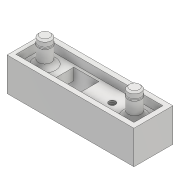
# Autodesk Inventor part: sipmHolder
Saved by Autodesk Inventor 2018 (Build 220112000, 112)
## iProperties
Created: 2017-05-10
Part Number: sipmHolder
Material: ABS Plastic
Document SubType Name: Modeling
Designer: sawaiz
Density: 1.06 g/cm^3
Appearance: Smooth - White
Author: sawaiz
Autodesk Inventor part; units mm, degrees
ref_plane "YZ Plane" through (0, 0, 0) normal (1, 0, 0) x (0, 1, 0)
sketch "Sketch1" plane through (0, 0, 0) normal (0, 0, 1) x (1, 0, 0)
  line L0 (-11.4, -3.5) -> (11.4, -3.5)
  line L1 (11.4, -3.5) -> (11.4, 3.5)
  line L2 (11.4, 3.5) -> (-11.4, 3.5)
  line L3 (-11.4, 3.5) -> (-11.4, -3.5)
  line L4 (-11.4, -3.5) -> (11.4, 3.5) construction
  line L5 (11.4, -3.5) -> (-11.4, 3.5) construction
  point P0 (0, 0)
  dimension "d0" = 22.8
  dimension "d1" = 7
  constraints: 12 end point, 2 midpoint, 2 parallel, 1 horizontal, 1 perpendicular
  measures "d0" distance of L2.end L1.end
  measures "d1" distance of L1.end L0.end
extrude "Extrusion1" add sketch "Sketch1" along normal mid plane 6
sketch "Sketch2" plane through (0, 0, 3) normal (0, 0, 1) x (1, 0, 0)
  line L0 (-5, 2.1) -> (-0.5, 2.1)
  line L1 (-0.5, 2.1) -> (-0.5, -2.1)
  line L2 (-0.5, -2.1) -> (-5, -2.1)
  line L3 (-5, -2.1) -> (-5, 2.1)
  line L4 (-5, 2.1) -> (-0.5, -2.1) construction
  line L5 (-0.5, 2.1) -> (-5, -2.1) construction
  line L6 (-11.4, 3.5) -> (-11.4, -3.5) projected
  line L7 (-2.75, 0) -> (-11.4, 0) construction
  point P0 (0, 0)
  dimension "d4" = 4.2
  dimension "d5" = 4.5
  dimension "d6" = 6.4
  constraints: 14 end point, 3 midpoint, 2 horizontal, 2 parallel, 1 perpendicular
  measures "d4" distance of L0.end L1.end
  measures "d5" distance of L0.start L0.end
  measures "d6" distance between parallel lines of L6 L3
extrude "Extrusion2" cut sketch "Sketch2" against normal through all
sketch "Sketch3" plane through (0, 0, 3) normal (0, 0, 1) x (1, 0, 0)
  line L0 (-5, -2.1) -> (-5, 2.1) projected
  line L1 (-5, 2.1) -> (-0.5, 2.1) projected
  line L2 (-0.5, 2.1) -> (-0.5, -2.1) projected
  line L3 (-0.5, -2.1) -> (-5, -2.1) projected
  line L4 (-11.4, -3.5) -> (11.4, -3.5) projected
  line L5 (11.4, -3.5) -> (11.4, 3.5) projected
  line L6 (11.4, 3.5) -> (-11.4, 3.5) projected
  line L7 (-11.4, 3.5) -> (-11.4, -3.5) projected
  line L8 (-10.7, -2.6) -> (10.5, -2.6)
  line L9 (10.5, -2.6) -> (10.5, 2.6)
  line L10 (10.5, 2.6) -> (-10.7, 2.6)
  line L11 (-10.7, 2.6) -> (-10.7, -2.6)
  line L12 (-10.7, -2.6) -> (10.5, 2.6) construction
  line L13 (10.5, -2.6) -> (-10.7, 2.6) construction
  dimension "d11" = 0.7
  dimension "d12" = 0.9
  dimension "d13" = 5.2
  dimension "d14" = 21.2
  constraints: 12 end point, 2 parallel, 1 horizontal, 1 perpendicular
  measures "d11" distance between parallel lines of L7 L11
  measures "d12" distance between parallel lines of L6 L10
  measures "d13" distance of L10.end L8.start
  measures "d14" distance of L9.end L10.end
extrude "Extrusion3" cut sketch "Sketch3" against normal blind 1.5 contours L11 L10 L9 L8
sketch "Sketch4" plane through (0, 0, -3) normal (0, 0, -1) x (-1, 0, 0)
  line L0 (-2.6, -2.1) -> (5, -2.1)
  line L1 (5, -2.1) -> (5, 2.1)
  line L2 (5, 2.1) -> (-2.6, 2.1)
  line L3 (-2.6, 2.1) -> (-2.6, -2.1)
  line L4 (-2.6, -2.1) -> (5, 2.1) construction
  line L5 (5, -2.1) -> (-2.6, 2.1) construction
  line L6 (5, 2.1) -> (5, -2.1) projected
  line L7 (5, -2.1) -> (0.5, -2.1) projected
  line L8 (0.5, -2.1) -> (0.5, 2.1) projected
  line L9 (0.5, 2.1) -> (5, 2.1) projected
  line L10 (-11.4, -3.5) -> (11.4, -3.5) projected
  line L11 (11.4, -3.5) -> (11.4, 3.5) projected
  line L12 (11.4, 3.5) -> (-11.4, 3.5) projected
  line L13 (-11.4, 3.5) -> (-11.4, -3.5) projected
  line L14 (0.5, 2.1) -> (5, 2.1) projected
  line L15 (5, -2.1) -> (0.5, -2.1) projected
  line L16 (5, 2.1) -> (5, -2.1) projected
  point P0 (0, 0)
  point P1 (1.2, 0)
  dimension "d17" = 14
  constraints: 12 end point, 3 collinear, 2 midpoint, 2 parallel, 1 horizontal, 1 perpendicular
  measures "d17" distance between parallel lines of L11 L3
extrude "Extrusion4" cut sketch "Sketch4" against normal blind 2.9 contours L3 L2 L8 L0 | L8 L2 L1 L0
sketch "Sketch5" plane through (0, 0, -3) normal (0, 0, -1) x (-1, 0, 0)
  line L0 (6.4, -2.1) -> (-6.5, -2.1)
  line L1 (-6.5, -2.1) -> (-6.5, 2.1)
  line L2 (-6.5, 2.1) -> (6.4, 2.1)
  line L3 (6.4, 2.1) -> (6.4, -2.1)
  line L4 (6.4, -2.1) -> (-6.5, 2.1) construction
  line L5 (-6.5, -2.1) -> (6.4, 2.1) construction
  line L6 (-2.6, 2.1) -> (5, 2.1) projected
  line L7 (5, -2.1) -> (-2.6, -2.1) projected
  line L8 (11.4, -3.5) -> (11.4, 3.5) projected
  point P0 (0, 0)
  point P1 (-0.05, 0)
  dimension "d20" = 12.9
  dimension "d21" = 5
  constraints: 12 end point, 2 collinear, 2 midpoint, 2 parallel, 1 horizontal, 1 perpendicular
  measures "d20" distance of L1.end L2.end
  measures "d21" distance between parallel lines of L8 L3
extrude "Extrusion5" cut sketch "Sketch5" against normal blind 2.4
sketch "Sketch6" plane through (0, 0, -3) normal (0, 0, -1) x (-1, 0, 0)
  line L0 (-6.5, 2.1) -> (6.4, 2.1) projected
  line L1 (6.4, 2.1) -> (6.4, -2.1) projected
  line L2 (6.4, -2.1) -> (-6.5, -2.1) projected
  line L3 (-6.5, -2.1) -> (-6.5, 2.1) projected
  line L4 (-11.4, -3.5) -> (11.4, -3.5) projected
  line L5 (11.4, -3.5) -> (11.4, 3.5) projected
  line L6 (11.4, 3.5) -> (-11.4, 3.5) projected
  line L7 (-11.4, 3.5) -> (-11.4, -3.5) projected
  point P0 (0, 0)
  constraints: 4 coincident
hole "Hole1" at (-6.4, 2.1, -3) at (-6.4, -2.1, -3) at (6.5, -2.1, -3) at (6.5, 2.1, -3) direction (0, 0, 1) diameter 0.5 depth 2.4
sketch "Sketch7" plane through (0, 0, -3) normal (0, 0, -1) x (-1, 0, 0)
  line L0 (-11.4, -3.5) -> (11.4, -3.5) projected
  line L1 (11.4, -3.5) -> (11.4, 3.5) projected
  line L2 (11.4, 3.5) -> (-11.4, 3.5) projected
  line L3 (-11.4, 3.5) -> (-11.4, -3.5) projected
  arc A0 (-6.5, -1.85) -> (-6.25, -2.1) centre (-6.5, -2.1) ccw projected
  line L4 (-6.5, -1.85) -> (-6.5, 1.85) projected
  arc A1 (-6.25, 2.1) -> (-6.5, 1.85) centre (-6.5, 2.1) ccw projected
  line L5 (-6.25, 2.1) -> (6.15, 2.1) projected
  arc A2 (6.4, 1.85) -> (6.15, 2.1) centre (6.4, 2.1) ccw projected
  line L6 (6.4, 1.85) -> (6.4, -1.85) projected
  arc A3 (6.15, -2.1) -> (6.4, -1.85) centre (6.4, -2.1) ccw projected
  line L7 (6.15, -2.1) -> (-6.25, -2.1) projected
  line L8 (-6.5, -1.85) -> (-6.5, 1.85) projected
  line L9 (-11.4, 3.5) -> (-11.4, -3.5) projected
  line L10 (11.4, -3.5) -> (11.4, 3.5) projected
  line L11 (6.4, 1.85) -> (6.4, -1.85) projected
  arc A4 (9.4189, -0.0387) -> (6.4, 2.1) centre (6.4, -1.1) ccw
  arc A5 (8.4755, -0.3703) -> (6.4, 1.1) centre (6.4, -1.1) ccw
  arc A6 (9.4189, -0.0387) -> (11.4, -1.4422) centre (11.4, 0.6578) ccw
  arc A7 (8.4755, -0.3703) -> (11.4, -2.4422) centre (11.4, 0.6578) ccw
  line L12 (6.4, 1.1) -> (6.4, 2.1)
  line L13 (11.4, -2.4422) -> (11.4, -1.4422)
  line L14 (11.4, 3.5) -> (11.4, -3.5) projected
  point P0 (0, 0)
  dimension "d36" = 1
  dimension "d37" = 2.2
  dimension "d38" = 2.1
  constraints: 8 point on circle, 4 centre point, 4 end point, 3 point on line, 2 collinear, 2 concentric, 2 line through centre, 2 tangent
  measures "d36" radial gap between concentric circles of A4 A5
  measures "d37" radius of A5
  measures "d38" radius of A6
extrude "Extrusion7" cut sketch "Sketch7" against normal blind 1.5 contours A7 A5 L6 A2 A4 A6 L1 | A2 L12 A4
sketch "Sketch8" plane through (0, 0, -0.6) normal (0, 0, -1) x (-1, 0, 0)
  line L0 (11.4, 3.5) -> (-11.4, 3.5) projected
  line L1 (11.4, -3.5) -> (11.4, -2.4422) projected
  point P0 (0, 0)
  point P1 (-4, 0)
  dimension "d41" = 3.5
  dimension "d42" = 15.4
  measures "d41" distance from line of L0 point (-4, 0)
  measures "d42" distance from line of L1 point (-4, 0)
hole "Hole2" at (4, 0, -0.6) direction (0, 0, 1) diameter 1.181 end through all thread size "0-80 UNF" class "2B" standard "ANSI Unified Screw Threads"
sketch "Sketch9" plane through (0, 0, 1.5) normal (0, 0, 1) x (1, 0, 0)
  circle A0 centre (-8.1, 0) radius 1.15
  circle A1 centre (8, 0) radius 1.15
  line L0 (-8.1, 0) -> (8, 0) construction
  line L1 (11.4, 3.5) -> (-11.4, 3.5) projected
  line L2 (-11.4, 3.5) -> (-11.4, -3.5) projected
  point P0 (0, 0)
  dimension "d50" = 3.5
  dimension "d51" = 16.1
  dimension "d52" = 3.3
  dimension "d53" = 2.3
  constraints: 2 centre point, 2 end point, 1 equal radius, 1 horizontal
  measures "d50" distance between parallel lines of L1 L0
  measures "d51" distance of L0.start L0.end
  measures "d52" distance from line of L2 L0.start
  measures "d53" diameter of A0
extrude "Extrusion8" add sketch "Sketch9" along normal blind 4.5
chamfer "Chamfer1" distance 0.3 angle 45 2 edges at (-9.25, 0, 6) (6.85, 0, 6)
ref_plane "Work Plane1" through (-8.1, 0, 4.8) normal (0, 0, 1) x (1, 0, 0)
sketch "Sketch10" plane through (-8.1, 0, 4.8) normal (0, 0, 1) x (1, 0, 0)
  circle A0 centre (0, 0) radius 1.15 projected
  circle A1 centre (16.1, 0) radius 1.15 projected
  circle A2 centre (0, 0) radius 1.2
  circle A3 centre (16.1, 0) radius 1.2
  point P0 (8.1, 0)
  dimension "d60" = 2.4
  dimension "d61" = 2.4
  constraints: 2 centre point, 2 coincident
  measures "d60" diameter of A2
  measures "d61" diameter of A3
extrude "Extrusion9" add sketch "Sketch10" against normal blind 0.2
ref_plane "Work Plane2" through (-11.4, 0, 3) normal (0, -1, 0) x (1, 0, 0)
sketch "Sketch11" plane through (-11.4, 0, 3) normal (0, -1, 0) x (1, 0, 0)
  line L0 (4.45, 2.7) -> (2.15, 2.7) projected
  line L1 (4.45, 1.8) -> (2.15, 1.8) projected
  line L2 (2.1, 1.6) -> (4.5, 1.6) projected
  line L3 (2.1, 1.8) -> (4.5, 1.8) projected
  line L4 (2.15, 1.6) -> (4.45, 1.6) projected
  line L5 (2.15, -1.5) -> (4.45, -1.5) projected
  line L6 (20.55, 2.7) -> (18.25, 2.7) projected
  line L7 (20.55, 1.8) -> (18.25, 1.8) projected
  line L8 (18.2, 1.6) -> (20.6, 1.6) projected
  line L9 (18.2, 1.8) -> (20.6, 1.8) projected
  line L10 (18.25, 1.6) -> (20.55, 1.6) projected
  line L11 (18.25, -1.5) -> (20.55, -1.5) projected
  line L12 (2.1, 1.8) -> (4.5, 1.8) projected
  line L13 (2.1, 1.8) -> (2.15, 1.9374)
  line L14 (2.1, 1.6) -> (2.15, 1.55)
  line L15 (2.15, -1.5) -> (2.15, 1.6) projected
  line L16 (2.15, 1.8) -> (2.15, 2.7) projected
  line L17 (2.15, 1.9374) -> (2.15, 1.8)
  line L18 (2.1, 1.8) -> (2.15, 1.8)
  line L19 (2.15, 1.55) -> (2.15, 1.6)
  line L20 (2.1, 1.6) -> (4.5, 1.6) projected
  line L21 (2.1, 1.6) -> (2.15, 1.6)
  line L22 (2.45, 3) -> (4.15, 3) projected
  line L23 (3.3, 3) -> (3.3, 1.6)
  line L24 (2.15, 1.6) -> (4.45, 1.6) projected
  point P0 (11.4, -3)
  dimension "d68" = 20
  dimension "d69" = 45
  constraints: 14 end point, 4 point on line, 2 midpoint, 1 collinear, 1 vertical
  measures "d68" angle of L16 L13
  measures "d69" angle of L15 L14
revolve "Revolution1" add sketch "Sketch11" angle 360 about axis through (-8.1, 0, 6) along (0, 0, -1) contours L15 L14 L2 | L16 L3 L13
sketch "Sketch12" plane through (-11.4, 0, 3) normal (0, -1, 0) x (1, 0, 0)
  line L0 (18.25, 1.8) -> (18.25, 2.7) projected
  line L1 (18.2, 1.8) -> (20.6, 1.8) projected
  line L2 (18.2, 1.8) -> (18.2, 1.6) projected
  line L3 (18.25, -1.5) -> (18.25, 1.6) projected
  line L4 (18.2, 1.6) -> (20.6, 1.6) projected
  line L5 (20.6, 1.8) -> (20.6, 1.6) projected
  line L6 (20.55, 1.8) -> (20.55, 2.7) projected
  line L7 (20.55, -1.5) -> (20.55, 1.6) projected
  line L8 (18.2, 1.8) -> (18.25, 1.9374)
  line L9 (20.55, 1.8) -> (18.25, 1.8) projected
  line L10 (18.25, 1.8) -> (18.25, 1.9374)
  line L11 (18.25, 1.8) -> (18.2, 1.8)
  line L12 (18.25, 1.55) -> (18.2, 1.6)
  line L13 (18.25, 1.6) -> (20.55, 1.6) projected
  line L14 (18.25, 1.6) -> (18.2, 1.6)
  line L15 (18.25, 1.6) -> (18.25, 1.55)
  line L16 (18.55, 3) -> (20.25, 3) projected
  line L17 (19.4, 3) -> (19.4, 1.6)
  point P0 (11.4, -3)
  dimension "d71" = 70
  dimension "d72" = 45
  constraints: 14 end point, 2 collinear, 2 midpoint, 2 perpendicular, 2 point on line
  measures "d71" angle of L11 L8
  measures "d72" angle of L15 L12
revolve "Revolution2" add sketch "Sketch12" angle 360 about axis through (8, 0, 6) along (0, 0, -1) contours L1 L8 L0 | L4 L3 L12
fillet "Fillet1" radius 0.8 2 edges at (-9.25, 0, 1.5) (6.85, 0, 1.5)
body "Solid1"
